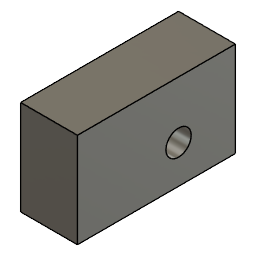
T-H04 (Autodesk Fusion 360 design; units mm, degrees)
Autodesk Fusion 360 part; units mm, degrees
sketch "草图1" plane through (0, 0, 0) normal (1, 0, 0) x (0, 0, -1)
  line L0 (0, 0) -> (50, 0)
  line L1 (50, 0) -> (50, 30)
  line L2 (50, 30) -> (0, 30)
  line L3 (0, 30) -> (0, 0)
  dimension "d1" = 50
  dimension "d2" = 30
  constraint horizontal L0
  constraint vertical L1
  constraint horizontal L2
  constraint vertical L3
  constraint coincident L0.start L3.end
  measures "d1" distance of L0.start L0.end
  measures "d2" distance of L0.end L1.end
extrude "拉伸1" add sketch "草图1" along normal blind 18
sketch "草图2" plane through (18, 0, 0) normal (1, 0, 0) x (0, 0, -1)
  line L0 (0, 30) -> (0, 0)
  line L1 (0, 0) -> (50, 0)
  line L2 (50, 0) -> (50, 30)
  line L3 (50, 30) -> (0, 30)
  line L4 (0, 0) -> (32, 0) construction
  line L5 (32, 0) -> (32, 12) construction
  circle A0 centre (32, 12) radius 4
  dimension "d5" = 32
  dimension "d6" = 12
  dimension "d7" = 8
  constraint coincident L0.end L1.start
  constraint perpendicular L0 L4
  constraint perpendicular L4 L5
  constraint coincident L5.end A0.centre
  measures "d5" distance of L0.end L4.end
  measures "d6" distance of L4.end L5.end
  measures "d7" diameter of A0
extrude "拉伸2" cut sketch "草图2" against normal through all contours A0
